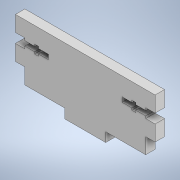
# Autodesk Inventor part: Крепление_мотора3_платформа
Saved by Autodesk Inventor 2020 (Build 240168000, 168)
## iProperties
Created: 2022-02-01
Part Number: Крепление_мотора3_платформа
Material: Типовые
Document SubType Name: Modeling
Designer: Администратор
Density: 1 g/cm^3
Appearance: По умолчанию
Autodesk Inventor part; units mm, degrees
ref_plane "YZ Plane" through (0, 0, 0) normal (1, 0, 0) x (0, 1, 0)
ref_plane "XZ Plane" through (0, 0, 0) normal (0, 1, 0) x (-1, 0, 0)
ref_plane "XY Plane" through (0, 0, 0) normal (0, 0, 1) x (1, 0, 0)
sketch "0" plane through (0, 0, 0) normal (0, 0, 1) x (1, 0, 0)
  line L0 (-44.5, -5) -> (-44.5, 5)
  line L1 (-44.5, 5) -> (-38.5, 5)
  line L2 (-38.5, 11) -> (-38.5, 9.5)
  line L3 (-38.5, 9.5) -> (-32.25, 9.5)
  line L4 (-23.5, 9.5) -> (-23.5, 6.5)
  line L5 (-23.5, 6.5) -> (-29.75, 6.5)
  line L6 (-32.25, 5.25) -> (-32.25, 6.5)
  line L7 (-32.25, 10.75) -> (-29.75, 10.75)
  line L8 (-29.75, 10.75) -> (-29.75, 9.5)
  line L9 (-29.75, 5.25) -> (-32.25, 5.25)
  line L10 (-32.25, 6.5) -> (-38.5, 6.5)
  line L11 (-29.75, 6.5) -> (-29.75, 5.25)
  line L12 (-32.25, 9.5) -> (-32.25, 10.75)
  line L13 (-38.5, 6.5) -> (-38.5, 5)
  line L14 (-44.5, 11) -> (-44.5, 21)
  line L15 (-38.5, 11) -> (-44.5, 11)
  line L16 (-44.5, 21) -> (-38.5, 21)
  line L17 (-29.75, 9.5) -> (-23.5, 9.5)
  line L18 (38.5, 21) -> (44.5, 21)
  line L19 (44.5, 21) -> (44.5, 11)
  line L20 (44.5, 11) -> (38.5, 11)
  line L21 (38.5, 5) -> (38.5, 6.5)
  line L22 (38.5, 6.5) -> (32.25, 6.5)
  line L23 (23.5, 6.5) -> (23.5, 9.5)
  line L24 (23.5, 9.5) -> (29.75, 9.5)
  line L25 (32.25, 10.75) -> (32.25, 9.5)
  line L26 (32.25, 5.25) -> (29.75, 5.25)
  line L27 (29.75, 5.25) -> (29.75, 6.5)
  line L28 (29.75, 10.75) -> (32.25, 10.75)
  line L29 (32.25, 9.5) -> (38.5, 9.5)
  line L30 (29.75, 9.5) -> (29.75, 10.75)
  line L31 (32.25, 6.5) -> (32.25, 5.25)
  line L32 (38.5, 9.5) -> (38.5, 11)
  line L33 (44.5, 5) -> (44.5, -5)
  line L34 (38.5, 5) -> (44.5, 5)
  line L35 (29.75, 6.5) -> (23.5, 6.5)
  line L36 (-38.5, 21) -> (38.5, 21)
  line L37 (38.5, -15) -> (13, -15)
  line L38 (13, -15) -> (13, -21)
  line L39 (-13, -21) -> (-13, -15)
  line L40 (-13, -15) -> (-38.5, -15)
  line L41 (-13, -21) -> (13, -21)
  line L42 (-44.5, -5) -> (-38.5, -5)
  line L43 (-38.5, -5) -> (-38.5, -15)
  line L44 (44.5, -5) -> (38.5, -5)
  line L45 (38.5, -5) -> (38.5, -15)
  constraints: 92 end point
extrude "Выдавливание1" add sketch "0" along normal blind 6
